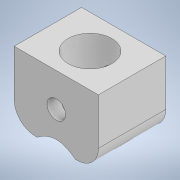
# Autodesk Inventor part: pist-dolni
Saved by Autodesk Inventor 2022 (Build 260153000, 153)
## iProperties
Created: 2022-11-09
Part Number: pist-dolni
Material: Generic
Document SubType Name: Modeling
Designer: matys
Density: 1 g/cm^3
Appearance: Default
Author: matys
Autodesk Inventor part; units mm, degrees
ref_plane "YZ Plane" through (0, 0, 0) normal (1, 0, 0) x (0, 1, 0)
ref_plane "XZ Plane" through (0, 0, 0) normal (0, 1, 0) x (-1, 0, 0)
ref_plane "XY Plane" through (0, 0, 0) normal (0, 0, 1) x (1, 0, 0)
sketch "Sketch1" plane through (0, 0, 0) normal (0, 1, 0) x (-1, 0, 0)
  line L0 (0, 0) -> (0, -10)
  line L1 (0, -10) -> (10, -10)
  line L2 (10, -10) -> (10, 0)
  line L3 (10, 0) -> (0, 0)
  dimension "d0" = 10
  dimension "d1" = 10
  constraints: 8 end point, 3 perpendicular, 1 vertical
  measures "d0" distance of L0.start L0.end
  measures "d1" distance of L0.end L1.end
extrude "Extrusion1" add sketch "Sketch1" along normal blind 8
sketch "Sketch2" plane through (0, 8, 0) normal (0, 1, 0) x (1, 0, 0)
  line L0 (-10, 10) -> (-10, 0) projected
  line L1 (-10, 0) -> (0, 0) projected
  line L2 (-10, 10) -> (0, 0)
  line L3 (0, 0) -> (-10, 0)
  line L4 (-10, 0) -> (0, 10)
  circle A0 centre (-5, 5) radius 2.6
  dimension "d4" = 5.2
  constraints: 6 end point, 1 centre point, 1 collinear, 1 midpoint, 1 perpendicular
  measures "d4" diameter of A0
extrude "Extrusion2" cut sketch "Sketch2" against normal through all contours A0 L4 L2 | L2 L4 A0 | L4 L2 A0 | L4 A0 L2
chamfer "Chamfer1" distance 2 distance2 3 1 edges at (-7.6, 0, -5) measured on face at (-8.1, 0, -5)
sketch "Sketch3" plane through (-10, 0, 0) normal (0, 0, 1) x (1, 0, 0)
  line L0 (7.6, 8) -> (7.6, 3) projected
  line L1 (7.6, 8) -> (10, 8)
  line L2 (10, 8) -> (10, 0)
  line L3 (10, 0) -> (7.6, 0)
  line L4 (0, 0) -> (10, 0) projected
  line L5 (2.4, 8) -> (7.6, 8) projected
  line L6 (7.6, 8) -> (7.6, 0)
  line L7 (0, 8) -> (10, 8) projected
  line L8 (10, 0) -> (10, 8) projected
  line L9 (0, 8) -> (10, 0)
  line L10 (10, 0) -> (0, 0)
  line L11 (10, 8) -> (0, 0)
  circle A0 centre (5, 4) radius 1.1
  dimension "d10" = 2.2
  constraints: 14 end point, 3 perpendicular, 2 point on line, 1 centre point, 1 horizontal, 1 midpoint
  measures "d10" diameter of A0
extrude "Extrusion3" cut sketch "Sketch3" against normal through all contours A0 L9 L11 | L11 L9 A0 | L11 A0 L9 | L9 A0 L11
fillet "Fillet1" radius 2.5 2 edges at (0, 0, -5) (-10, 0, -5)
sketch "Sketch4" plane through (0, 8, 0) normal (0, 1, 0) x (1, 0, 0)
  arc A0 (-4.5417, 2.4407) -> (-4.5417, 7.5593) centre (-5, 5) ccw projected
  line L0 (-5, 5) -> (0, 5)
  line L1 (0, 0) -> (0, 10) projected
  line L2 (0, 5) -> (0, 8)
  line L3 (0, 8) -> (-10, 8)
  line L4 (-10, 10) -> (-10, 0) projected
  line L5 (-10, 8) -> (-10, 0)
  line L6 (-10, 0) -> (0, 0)
  line L7 (0, 0) -> (0, 8)
  line L8 (0, 10) -> (-10, 10) projected
  line L9 (0, 8) -> (0, 10)
  line L10 (0, 10) -> (-10, 10)
  line L11 (-10, 10) -> (-10, 8)
  line L12 (-10, 0) -> (-10, 0)
  line L13 (0, 0) -> (-2.5, 0) projected
  line L14 (-10, 0) -> (0, 0)
  line L15 (0, 0) -> (0, 0)
  line L16 (-10, 0) -> (-10, 10) projected
  line L17 (-10, 5) -> (-10, 9)
  line L18 (-10, 9) -> (-10, 1)
  line L19 (-10, 1) -> (0, 1)
  line L20 (0, 10) -> (0, 0) projected
  line L21 (-10, 9) -> (0, 9)
  point P0 (0, 0)
  point P1 (-10, 0)
  dimension "d14" = 3
  dimension "d15" = 8
  dimension "d18" = 8
  constraints: 32 end point, 6 perpendicular, 6 point on line, 4 collinear, 3 midpoint, 1 vertical
  measures "d14" distance of L0.end L2.end
  measures "d15" distance of L3.end L5.end
  measures "d18" distance of L17.end L18.end
extrude "Extrusion4" cut sketch "Sketch4" against normal through all contours L6 L4 L19 L1 | L21 L4 L8 L1
body "Solid1"
